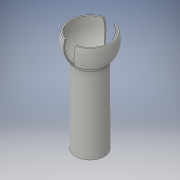
# Autodesk Inventor part: Castor(Chimpmunk)
Saved by Autodesk Inventor 2016 (Build 200138000, 138)
## iProperties
Created: 2016-10-13
Part Number: Castor(Chimpmunk)
Material: Generic
Document SubType Name: Modeling
Designer: brandn
Density: 1 g/cm^3
Appearance: Default
Author: brandn
Autodesk Inventor part; units mm, degrees
sketch "Sketch1" plane through (0, 0, 0) normal (0, 1, 0) x (-1, 0, 0)
  circle A0 centre (0, 0) radius 6.1665
  constraints: 1 centre point, 1 coincident
extrude "Extrusion1" add sketch "Sketch1" against normal blind 33.02
sketch "Sketch2" plane through (0, -33.02, 0) normal (0, -1, 0) x (1, 0, 0)
  point P0 (0, 0)
sketch "Sketch3" plane through (0, -33.02, 0) normal (0, -1, 0) x (1, 0, 0)
  point P0 (0, 0)
sketch "Sketch4" plane through (0, -33.02, 0) normal (0, -1, 0) x (1, 0, 0)
  point P0 (0, 0)
sketch "Sketch5" plane through (0, 0, 0) normal (0, 1, 0) x (1, 0, 0)
  point P0 (0, 0)
ref_plane "Work Plane1" through (0, 7.62, 0) normal (0, 1, 0) x (-1, 0, 0)
sketch "Sketch6" plane through (0, 7.62, 0) normal (0, 1, 0) x (-1, 0, 0)
  circle A0 centre (0, 0) radius 6.1665 projected
  arc A1 (0, 9.398) -> (0, -9.398) centre (0, 0) ccw
  line L0 (0, 9.398) -> (0, -9.398)
  arc A2 (-8.7249, 0) -> (8.7249, 0) centre (0, 0) ccw
  line L1 (-8.7249, 0) -> (8.7249, 0)
  dimension "d26" = 1.651
  dimension "d3" = 18.796
  dimension "d5" = 17.4498
  constraints: 4 end point, 4 point on circle, 2 centre point, 2 coincident, 1 horizontal, 1 vertical
  measures "d3" diameter of A1
  measures "d5" diameter of A2
revolve "Revolution1" add sketch "Sketch6" angle 360 about axis through (0, 7.62, 9.398) along (0, 0, -1) picked at (-0.4574, 4.0595) picked at (-7.7476, -1.1045) picked at (-4.0595, -0.4574) contours L0 L1 A0 | A0 L1 A2 L0 A1 | L0 A2 L1 A0 | A0 L1 L0
sketch "Sketch7" plane through (0, 7.62, 0) normal (0, 1, 0) x (-1, 0, 0)
  arc A0 (8.89, 0) -> (-8.89, 0) centre (0, 0) ccw
  line L0 (-8.89, 0) -> (8.89, 0)
  dimension "d6" = 17.78
  constraints: 2 end point, 2 point on circle, 1 centre point, 1 coincident
  measures "d6" diameter of A0
revolve "Revolution2" cut sketch "Sketch7" angle 360 about axis through (8.89, 7.62, 0) along (-1, 0, 0)
sketch "Sketch8" plane through (0, 0, 0) normal (0, 1, 0) x (-1, 0, 0)
  point P0 (0, 0)
ref_plane "Work Plane2" through (0, 10.668, 0) normal (0, 1, 0) x (-1, 0, 0)
sketch "Sketch9" plane through (0, 10.668, 0) normal (0, 1, 0) x (-1, 0, 0)
  line L0 (-10.2619, -10.332) -> (10.2619, -10.332)
  line L1 (10.2619, -10.332) -> (10.2619, 10.2385)
  line L2 (10.2619, 10.2385) -> (-10.2619, 10.2385)
  line L3 (-10.2619, 10.2385) -> (-10.2619, -10.332)
  point P0 (0, 0)
  constraints: 8 end point, 2 parallel, 1 horizontal, 1 perpendicular
extrude "Extrusion2" cut sketch "Sketch9" along normal blind 25.4
sketch "Sketch10" plane through (0, 0, 0) normal (0, 0, 1) x (1, 0, 0)
  line L0 (8.3512, 10.668) -> (-8.3512, 10.668) projected
  ellipse E0 centre (0, 10.668) end of major axis (-2.4361, 10.668) minor radius 9.1093
  point P0 (0, 0)
  constraints: 1 midpoint, 2 other
extrude "Extrusion3" cut sketch "Sketch10" along normal mid plane 25.4
sketch "Sketch11" plane through (0, -33.02, 0) normal (0, -1, 0) x (1, 0, 0)
  circle A0 centre (0, 0) radius 2.9972
  dimension "d13" = 5.9944
  constraints: 1 centre point, 1 coincident
  measures "d13" diameter of A0
ref_plane "Work Plane3" through (0, -30.7848, 0) normal (0, -1, 0) x (1, 0, 0)
sketch "Sketch13" plane through (0, 0, 0) normal (1, 0, 0) x (0, 1, 0)
  point P0 (0, 0)
ref_plane "Work Plane4" through (0, 0, 0) normal (1, 0, 0) x (0, 1, 0)
sketch "Sketch14" plane through (0, 0, 0) normal (1, 0, 0) x (0, 1, 0)
  line L0 (-33.02, 6.1665) -> (-33.02, -6.1665) projected
  line L1 (-33.02, 0) -> (-33.02, 2.9972)
  line L2 (-33.02, 0) -> (-26.67, 0)
  line L3 (-26.67, 0) -> (-26.67, 2.8702)
  line L4 (0, 6.1665) -> (-33.02, 6.1665) projected
  line L5 (-26.67, 2.8702) -> (-28.321, 2.8702)
  line L6 (-28.321, 2.8702) -> (-33.02, 2.9972)
  point P0 (0, 0)
  dimension "d23" = 2.9972
  dimension "d24" = 6.35
  dimension "d25" = 2.8702
  dimension "d26" = 1.651
  constraints: 10 end point, 2 perpendicular, 1 horizontal, 1 midpoint, 1 point on line
  measures "d23" distance of L1.start L1.end
  measures "d24" distance of L1.start L2.end
  measures "d25" distance of L2.end L3.end
  measures "d26" distance of L3.end L5.end
revolve "Revolution3" cut sketch "Sketch14" angle 360 about axis through (0, -33.02, 0) along (0, 1, 0)
fillet "Fillet1" radius 3.175 1 edges at (0, 0, -5.5007)
body "Solid1"
